test_2 (Autodesk Fusion 360 design; units mm, degrees)
Autodesk Fusion 360 part; units mm, degrees
note: some values were not read from the file. Chosen so that the rebuilt part matches the saved one: which bodies a step acts on.
sketch "Sketch1" plane through (0, 0, 0) normal (0, 1, 0) x (1, 0, 0)
  line L0 (0, 0) -> (-20, 0)
  line L1 (-20, 0) -> (-20, -60)
  line L2 (-20, -60) -> (0, -60)
  line L3 (0, -60) -> (0, 0)
  line L4 (0, -30) -> (-20, -30)
  line L5 (-10, 0) -> (-10, -60)
  line L6 (-13.8105, 0) -> (-18.9844, -8.9615)
  line L7 (-12.4249, -4.2) -> (-6.1895, -15)
  line L8 (-10, -15) -> (-12.1532, -11.2706)
  line L9 (-12.4249, -4.2) -> (-10, 0)
  line L10 (0, -15) -> (-20, -15)
  arc A0 (-18.9844, -8.9615) -> (-12.1532, -11.2706) centre (-15.8, -10.8) ccw
  circle A1 centre (-15.8, -10.8) radius 0.3771
  line L11 (-12.1532, -11.2706) -> (-16.2354, -4.2)
  line L12 (-16.1265, -10.6115) -> (-14.3301, -7.5)
  line L13 (-15.4414, -10.9166) -> (-14.3301, -7.5)
  dimension "d1" = 60
  dimension "d2" = 20
  dimension "d3" = 3.3
  dimension "d4" = 3.3
  dimension "d8" = 15
  dimension "d20" = 60
  dimension "d21" = 60
  dimension "d23" = 4.2
  dimension "d24" = 4.2
  constraint horizontal L0
  constraint vertical L1
  constraint horizontal L2
  constraint vertical L3
  constraint coincident L0.start L3.end
  constraint midpoint L3 L4.start
  constraint midpoint L1 L4.end
  constraint midpoint L0 L5.start
  constraint midpoint L2 L5.end
  constraint coincident L0 L6.start
  constraint coincident L0 L5.start
  constraint parallel L6 L9
  constraint parallel L7 L8
  constraint coincident L7.start L9.start
  constraint coincident L3 L10.start
  constraint coincident L1 L10.end
  constraint perpendicular L1 L10
  constraint coincident L5.start L9.end
  constraint midpoint L8.start L10
  constraint coincident L7.end L10
  constraint tangent L6 A0
  constraint concentric A0 A1
  constraint coincident L6 L11.end
  constraint parallel L8 L11
  constraint coincident A1 L12.start
  constraint coincident L11 L12.end
  constraint coincident A1 L13.start
  constraint collinear L9 L12
  constraint tangent A1 L12
  constraint tangent A1 L13
  measures "d1" distance of L0.start L2.end
  measures "d2" distance of L0.start L0.end
  measures "d3" distance of L6 L9
  measures "d4" distance of L7 L8
  measures "d8" distance of L4 L10
  measures "d20" angle of L8 L10
  measures "d21" angle of L0 L6
  measures "d23" distance of L10 A0.centre
  measures "d24" distance of L1 A0.centre
extrude "Extrude1" add sketch "Sketch1" along normal blind 5 contours L0 L3 L5 L7 L10 | L5 L7 L9 | L0 L1 L6 L8 L10 A0 | A1 L12 L13 | A1 makes body 1 at (-20, 1.6667, 5) makes body 2 at (-6.2048, 0, 6.4) makes body 3 at (-15.071, 1.6667, 9.7778)
ref_plane "WorkPlane1" through (-10, 0, 0) normal (1, 0, 0) x (0, 1, 0)
mirror "Mirror1" about plane through (-10, 0, 0) normal (1, 0, 0) of bodies 2 1 3 makes body 4 at (-4.929, 1.6667, 9.7778) makes body 5 at (0, 1.6667, 5) makes body 6 at (-13.7952, 0, 6.4)
move_body "Move1" bodies 4 6 5 to x (1, 0, 0) y (0, 1, 0) z (0, 0, 1) at (0, 0, 15)
pattern_linear "R-Pattern1" count 2 spacing 30 along (0, 0, 1) of bodies 6 5 2 1 3 4 makes body 7 at (-20, 1.6667, 35) makes body 8 at (-6.2048, 0, 36.4) makes body 9 at (-15.071, 3.3333, 39.7778) makes body 10 at (-4.929, 3.3333, 54.7778) makes body 11 at (0, 1.6667, 50) makes body 12 at (-13.7952, 0, 51.4)
equation "d4 = d3"
equation "d24 = d23"
